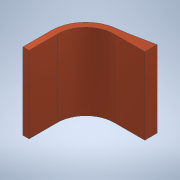
# Autodesk Inventor part: SoporteGoma
Saved by Autodesk Inventor 2022.2 (Build 262287010, 287A)
## iProperties
Created: 2022-03-28
Part Number: SoporteGoma
Material: Generic
Document SubType Name: Modeling
Designer: Santiago Larraín
Density: 1 g/cm^3
Appearance: Default
Author: Santiago Larraín
Autodesk Inventor part; units mm, degrees
ref_plane "YZ Plane" through (0, 0, 0) normal (1, 0, 0) x (0, 1, 0)
ref_plane "XZ Plane" through (0, 0, 0) normal (0, 1, 0) x (-1, 0, 0)
ref_plane "XY Plane" through (0, 0, 0) normal (0, 0, 1) x (1, 0, 0)
sketch "Sketch1" plane through (0, 0, 0) normal (0, 1, 0) x (-1, 0, 0)
  line L0 (0, 0) -> (20, 0)
  arc A0 (20, 0) -> (38.5, 18.5) centre (20, 18.5) ccw
  line L1 (38.5, 18.5) -> (38.5, 37)
  line L2 (38.5, 37) -> (42.5, 37)
  line L3 (42.5, 37) -> (42.5, 18.5)
  line L4 (0, 0) -> (0, -8)
  line L5 (20, -4) -> (0, -8)
  arc A1 (20, -4) -> (42.5, 18.5) centre (20, 18.5) ccw
  dimension "d0" = 20
  dimension "d3" = 18.5
  dimension "d4" = 4
  dimension "d5" = 8
  dimension "d6" = 4
  constraints: 12 end point, 4 point on circle, 2 centre point, 2 horizontal, 2 vertical, 1 coincident, 1 perpendicular
  measures "d0" distance of L0.start L0.end
  measures "d3" distance of L1.start L1.end
  measures "d4" distance of L1.end L2.end
  measures "d5" distance of L0.start L4.end
  measures "d6" distance of L0.end L5.start
extrude "Extrusion1" add sketch "Sketch1" along normal blind 50
chamfer "Chamfer1" distance 4.75 angle 45 1 edges at (-20, 25, -4)
body "Solid1"
